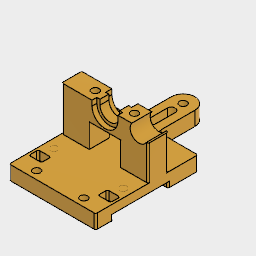
Extruder_Mount_F01 (Autodesk Fusion 360 design; units mm, degrees)
Autodesk Fusion 360 part; units mm, degrees
sketch "スケッチ1" plane through (0, 0, 0) normal (0, 0, 1) x (1, 0, 0)
  line L0 (27.5, 32.5) -> (-27.5, 32.5)
  line L1 (-27.5, 32.5) -> (-27.5, -32.5)
  line L2 (-27.5, -32.5) -> (27.5, -32.5)
  line L3 (27.5, -32.5) -> (27.5, 32.5)
  line L4 (27.5, 32.5) -> (-27.5, -32.5) construction
  line L5 (-27.5, 32.5) -> (27.5, -32.5) construction
  line L6 (-13, 32.5) -> (-13, 56.1)
  line L7 (-13, 56.1) -> (2, 56.1)
  line L8 (2, 56.1) -> (2, 32.5)
  circle A0 centre (-5.5, 56.1) radius 7.5
  line L9 (-5.5, 56.1) -> (-5.5, 32.5) construction
  circle A1 centre (-5.5, 36.1) radius 2.5
  circle A2 centre (-5.5, 48.6) radius 2.5
  line L10 (-3, 48.6) -> (-3, 36.1)
  line L11 (-8, 36.1) -> (-8, 48.6)
  line L12 (-27.5, 0.9) -> (27.5, 0.9)
  line L13 (27.5, 13.6) -> (-27.5, 13.6)
  dimension "d1" = 55
  dimension "d2" = 65
  dimension "d3" = 15
  dimension "d4" = 23.6
  dimension "d5" = 14.5
  dimension "d6" = 5
  dimension "d7" = 5
  dimension "d8" = 12.5
  dimension "d9" = 3.6
  dimension "d10" = 33.4
  dimension "d11" = 12.7
  measures "d1" distance of L1.end L2.end
  measures "d2" distance of L0.end L1.end
  measures "d3" distance of L6 L8
  measures "d4" distance of L0 L7
  measures "d5" distance of L1 L6
  measures "d6" diameter of A1
  measures "d7" diameter of A2
  measures "d8" distance of A1.centre A2.centre
  measures "d9" distance of L0 A1.centre
  measures "d10" distance of L2 L12
  measures "d11" distance of L12 L13
extrude "押し出し1" add sketch "スケッチ1" along normal blind 9 contours L0 L1 L3 L13 | L0 L6 L8 A0 A1 A2 L10 L11 | L1 L3 L12 L13 | L7 A0 A2 | L7 A0 | L1 L2 L3 L12
extrude "押し出し2" add sketch "スケッチ1" along normal blind 37 contours L1 L3 L12 L13
sketch "スケッチ2" plane through (0, 0, 0) normal (0, 0, -1) x (1, 0, 0)
  line L0 (-27.5, 32.5) -> (-27.5, -32.5)
  line L1 (-27.5, -32.5) -> (-13, -32.5)
  line L2 (-13, -32.5) -> (-13, -56.1)
  arc A0 (-13, -56.1) -> (2, -56.1) centre (-5.5, -56.1) ccw
  line L3 (2, -56.1) -> (2, -32.5)
  line L4 (2, -32.5) -> (27.5, -32.5)
  line L5 (27.5, -32.5) -> (27.5, 32.5)
  line L6 (27.5, 32.5) -> (-27.5, 32.5)
  arc A1 (-8, -48.6) -> (-3, -48.6) centre (-5.5, -48.6) ccw
  line L7 (-8, -48.6) -> (-8, -36.1)
  arc A2 (-3, -36.1) -> (-8, -36.1) centre (-5.5, -36.1) ccw
  line L8 (-3, -36.1) -> (-3, -48.6)
  line L9 (27.5, 21.5) -> (16.5, 21.5)
  line L10 (16.5, 21.5) -> (16.5, -13.5)
  line L11 (16.5, -13.5) -> (27.5, -13.5)
  line L12 (17.3, 6) -> (26.7, 6)
  line L13 (26.7, 6) -> (26.7, -6)
  line L14 (26.7, -6) -> (17.3, -6)
  line L15 (17.3, -6) -> (17.3, 6)
  line L16 (18, 21.5) -> (18, 15.5)
  line L17 (18, 15.5) -> (26, 15.5)
  line L18 (26, 15.5) -> (26, 21.5)
  circle A3 centre (22, 9.525) radius 2.35
  circle A4 centre (22, -9.525) radius 2.35
  line L19 (22, -13.5) -> (22, 21.5) construction
  line L20 (0, 32.5) -> (0, -32.5) construction
  line L21 (-16.5, -13.5) -> (-27.5, -13.5)
  line L22 (-16.5, 21.5) -> (-16.5, -13.5)
  line L23 (-27.5, 21.5) -> (-16.5, 21.5)
  line L24 (-18, 15.5) -> (-26, 15.5)
  line L25 (-18, 21.5) -> (-18, 15.5)
  line L26 (-26, 15.5) -> (-26, 21.5)
  circle A5 centre (-22, 9.525) radius 2.35
  line L27 (-17.3, 6) -> (-26.7, 6)
  line L28 (-26.7, 6) -> (-26.7, -6)
  line L29 (-17.3, -6) -> (-17.3, 6)
  line L30 (-26.7, -6) -> (-17.3, -6)
  circle A6 centre (-22, -9.525) radius 2.35
  circle A7 centre (0, 0) radius 2.35
  circle A8 centre (-12, -12) radius 1.5
  circle A9 centre (12, -12) radius 1.5
  circle A10 centre (12, 12) radius 1.5
  circle A11 centre (-12, 12) radius 1.5
  circle A12 centre (0, 0) radius 1.5
  dimension "d16" = 4.7
  dimension "d17" = 4.7
  dimension "d18" = 35
  dimension "d19" = 11
  dimension "d20" = 11
  dimension "d21" = 12
  dimension "d22" = 7.5
  dimension "d23" = 3.975
  dimension "d24" = 11.975
  dimension "d25" = 9.4
  dimension "d26" = 0.8
  dimension "d27" = 6
  dimension "d28" = 8
  dimension "d29" = 1.5
  dimension "d30" = 4.7
  dimension "d31" = 3
  dimension "d32" = 12
  dimension "d33" = 12
  dimension "d35" = 360
  dimension "d45" = 3
  measures "d16" diameter of A3
  measures "d17" diameter of A4
  measures "d18" distance of L9 L11
  measures "d19" distance of L6 L9
  measures "d20" distance of L10.end L11.end
  measures "d21" distance of L12.end L13.end
  measures "d22" distance of L11 L14
  measures "d23" distance of L11 A4.centre
  measures "d24" distance of L9 A3.centre
  measures "d25" distance of L13.end L14.end
  measures "d26" distance of L5 L13
  measures "d27" distance of L17.end L18.end
  measures "d28" distance of L16.end L17.end
  measures "d29" distance of L5 L18
  measures "d30" diameter of A7
  measures "d31" diameter of A8
  measures "d32" distance of A7.centre A8.centre
  measures "d33" distance of A7.centre A8.centre
  measures "d45" diameter of A12
extrude "押し出し3" cut sketch "スケッチ2" against normal through all contours L9 L16 L17 L18
extrude "押し出し4" cut sketch "スケッチ2" against normal blind 8.5 contours A3 | A4
extrude "押し出し5" cut sketch "スケッチ2" against normal blind 5 contours L12 L13 L14 L15
extrude "押し出し6" cut sketch "スケッチ2" against normal blind 3.5 contours L5 L9 L10 L11 L16 L17 L18
mirror "ミラー1" about plane through (0, 0, 0) normal (1, 0, 0) of "押し出し3", "押し出し4", "押し出し5", "押し出し6"
extrude "押し出し7" cut sketch "スケッチ2" against normal blind 8 contours A8 | A9 | A10 | A11
extrude "押し出し8" cut sketch "スケッチ2" against normal blind 8 contours A12
extrude "押し出し9" cut sketch "スケッチ2" against normal blind 5 contours A7
sketch "スケッチ3" plane through (0, 13.6, 0) normal (0, 1, 0) x (-1, 0, 0)
  line L0 (-27.5, 9) -> (27.5, 9)
  line L1 (27.5, 9) -> (27.5, 37)
  line L2 (27.5, 37) -> (-27.5, 37)
  line L3 (-27.5, 37) -> (-27.5, 9)
  line L4 (-10, 9) -> (-10, 24.2)
  line L5 (-10, 24.2) -> (10, 24.2)
  line L6 (10, 24.2) -> (10, 9)
  line L7 (0, 37) -> (0, 0) construction
  circle A0 centre (0, 33.75) radius 8.25
  circle A1 centre (0, 33.75) radius 6.25
  circle A2 centre (-21.5, 33.75) radius 5.5
  line L8 (6.25, 37) -> (6.25, 33.75)
  line L9 (-6.25, 37) -> (-6.25, 33.75)
  line L10 (8.25, 37) -> (8.25, 33.75)
  line L11 (-8.25, 37) -> (-8.25, 33.75)
  line L12 (-27.5, 31) -> (-26.2631, 31)
  line L13 (-27.5, 9) -> (-2, 9)
  line L14 (13, 9) -> (27.5, 9)
  circle A3 centre (10, 16.6) radius 1.25
  dimension "d50" = 16.5
  dimension "d51" = 12.5
  dimension "d52" = 11
  dimension "d53" = 3.25
  dimension "d54" = 6
  dimension "d55" = 3.25
  dimension "d56" = 22
  dimension "d57" = 20
  dimension "d58" = 17.5
  dimension "d59" = 15.2
  dimension "d60" = 2.5
  dimension "d61" = 7.6
  measures "d50" diameter of A0
  measures "d51" diameter of A1
  measures "d52" diameter of A2
  measures "d53" distance of L2 A0.centre
  measures "d54" distance of L3 A2.centre
  measures "d55" distance of L2 A2.centre
  measures "d56" distance of L12 L13
  measures "d57" distance of L4.end L5.end
  measures "d58" distance of L1 L6
  measures "d59" distance of L5.end L6.end
  measures "d60" diameter of A3
  measures "d61" distance of L0 A3.centre
extrude "押し出し10" cut sketch "スケッチ3" against normal through all contours L0 L4 L5 L6 L13 A3 | L6 A3 picked at (9.5938, 16.5073)
extrude "押し出し11" cut sketch "スケッチ3" against normal through all contours L2 A1 L9 | L2 A1 | L2 A1 L8 picked at (-0.4636, 33.8856)
extrude "押し出し12" cut sketch "スケッチ3" against normal through all from surface at -9.6 contours L2 A0 L11 | L2 A0 A1 L8 L9 | L2 A0 L10
extrude "押し出し13" cut sketch "スケッチ3" against normal blind 3.95 contours L2 A0 L11 | L2 A0 A1 L8 L9 | L2 A0 L10
extrude "押し出し14" cut sketch "スケッチ3" against normal through all contours L2 L3 A2 L12 | L2 A2 picked at (-22.8229, 31.257)
extrude "押し出し15" cut sketch "スケッチ3" against normal blind 4 contours L6 A3 picked at (10.7965, 16.3106)
sketch "スケッチ4" plane through (27.5, 0, 0) normal (1, 0, 0) x (0, 1, 0)
  line L0 (13.6, 31) -> (0.9, 31)
  line L1 (0.9, 31) -> (0.9, 9)
  line L2 (0.9, 9) -> (-32.5, 9)
  line L3 (-32.5, 9) -> (-32.5, 0)
  line L4 (-32.5, 0) -> (-21.5, 0)
  line L5 (-21.5, 0) -> (-21.5, 3.5)
  line L6 (-21.5, 3.5) -> (13.5, 3.5)
  line L7 (13.5, 3.5) -> (13.5, 0)
  line L8 (13.5, 0) -> (32.5, 0)
  line L9 (32.5, 0) -> (32.5, 9)
  line L10 (32.5, 9) -> (13.6, 9)
  line L11 (13.6, 9) -> (13.6, 31)
  circle A0 centre (13.6, 15.6) radius 1.25
  dimension "d71" = 2.5
  dimension "d72" = 6.6
  measures "d71" diameter of A0
  measures "d72" distance of L10.end A0.centre
extrude "押し出し16" cut sketch "スケッチ4" against normal blind 11 from surface at -3.5 contours L11 A0 picked at (13.1845, 15.9855)
sketch "スケッチ5" plane through (0, 0, 9) normal (0, 0, 1) x (-1, 0, 0)
  line L0 (-18, 15.5) -> (-26, 15.5)
  line L1 (-26, 15.5) -> (-26, 21.5)
  line L2 (-26, 21.5) -> (-18, 21.5)
  line L3 (-18, 21.5) -> (-18, 15.5)
  line L4 (27.5, -13.6) -> (10, -13.6)
  line L5 (10, -13.6) -> (10, -0.9)
  line L6 (10, -0.9) -> (27.5, -0.9)
  line L7 (27.5, -0.9) -> (27.5, 32.5)
  line L8 (27.5, 32.5) -> (-27.5, 32.5)
  line L9 (-27.5, 32.5) -> (-27.5, -0.9)
  line L10 (-27.5, -0.9) -> (-10, -0.9)
  line L11 (-10, -0.9) -> (-10, -13.6)
  line L12 (-10, -13.6) -> (-27.5, -13.6)
  line L13 (-27.5, -13.6) -> (-27.5, -32.5)
  line L14 (-27.5, -32.5) -> (-2, -32.5)
  line L15 (-2, -32.5) -> (-2, -56.1)
  arc A0 (-2, -56.1) -> (13, -56.1) centre (5.5, -56.1) ccw
  line L16 (13, -56.1) -> (13, -32.5)
  line L17 (13, -32.5) -> (27.5, -32.5)
  line L18 (27.5, -32.5) -> (27.5, -13.6)
  arc A1 (3, -48.6) -> (8, -48.6) centre (5.5, -48.6) ccw
  line L19 (3, -48.6) -> (3, -36.1)
  arc A2 (8, -36.1) -> (3, -36.1) centre (5.5, -36.1) ccw
  line L20 (8, -36.1) -> (8, -48.6)
  circle A3 centre (5.5, -56.1) radius 2.35
  circle A4 centre (5.5, -56.1) radius 1.75
  circle A5 centre (15, 27.5) radius 2.35
  circle A6 centre (15, 27.5) radius 1.75
  circle A7 centre (-15, 27.5) radius 2.35
  circle A8 centre (-15, 27.5) radius 1.75
  line L21 (18, 21.5) -> (26, 21.5)
  line L22 (26, 21.5) -> (26, 15.5)
  line L23 (26, 15.5) -> (18, 15.5)
  line L24 (18, 15.5) -> (18, 21.5)
  dimension "d76" = 4.7
  dimension "d77" = 3.5
  dimension "d78" = 4.7
  dimension "d79" = 3.5
  dimension "d80" = 4.7
  dimension "d81" = 3.5
  dimension "d82" = 5
  dimension "d83" = 12.5
  dimension "d84" = 12.5
  measures "d76" diameter of A3
  measures "d77" diameter of A4
  measures "d78" diameter of A5
  measures "d79" diameter of A6
  measures "d80" diameter of A7
  measures "d81" diameter of A8
  measures "d82" distance of L8 A5.centre
  measures "d83" distance of L7 A5.centre
  measures "d84" distance of L9 A7.centre
extrude "押し出し17" cut sketch "スケッチ5" against normal blind 8 contours A4 | A6 | A8
extrude "押し出し18" cut sketch "スケッチ5" against normal blind 5 contours A3 | A5 | A7
sketch "スケッチ6" plane through (0, 0, 37) normal (0, 0, 1) x (-1, 0, 0)
  line L0 (8.25, -9.65) -> (8.25, -13.6)
  line L1 (8.25, -13.6) -> (27.5, -13.6)
  line L2 (27.5, -13.6) -> (27.5, -0.9)
  line L3 (27.5, -0.9) -> (8.25, -0.9)
  line L4 (8.25, -0.9) -> (8.25, -4)
  line L5 (8.25, -4) -> (6.25, -4)
  line L6 (6.25, -4) -> (6.25, -9.65)
  line L7 (6.25, -9.65) -> (8.25, -9.65)
  line L8 (-27.5, -13.6) -> (-27.5, -0.9)
  line L9 (27.5, -7.25) -> (-27.5, -7.25) construction
  circle A0 centre (12.5, -7.25) radius 2.35
  circle A1 centre (12.5, -7.25) radius 1.75
  circle A2 centre (-12.5, -7.25) radius 2.35
  circle A3 centre (-12.5, -7.25) radius 1.75
  dimension "d89" = 4.7
  dimension "d90" = 4.7
  dimension "d91" = 3.5
  dimension "d92" = 3.5
  dimension "d93" = 15
  dimension "d94" = 15
  measures "d89" diameter of A0
  measures "d90" diameter of A2
  measures "d91" diameter of A3
  measures "d92" diameter of A1
  measures "d93" distance of L2 A0.centre
  measures "d94" distance of L8 A2.centre
extrude "押し出し19" cut sketch "スケッチ6" against normal blind 10 contours A1 | A3
extrude "押し出し20" cut sketch "スケッチ6" against normal blind 5 contours A0 | A2
fillet "フィレット1" radius 1 12 edges at (27.5, -32.5, 4.5) (27.5, -21.5, 1.75) (27.5, 13.5, 1.75) (27.5, 32.5, 4.5) (-27.5, 32.5, 4.5) (-27.5, -32.5, 4.5) (-27.5, 13.6, 23) (-27.5, 0.9, 23) (27.5, 0.9, 20) (27.5, 13.6, 20) (-27.5, 13.5, 1.75) (-27.5, -21.5, 1.75)
fillet "フィレット2" radius 1 8 edges at (18, -15.5, 6.25) (18, -21.5, 6.25) (26, -15.5, 6.25) (26, -21.5, 6.25) (-18, -21.5, 6.25) (-18, -15.5, 6.25) (-26, -15.5, 6.25) (-26, -21.5, 6.25)
fillet "フィレット3" radius 1 3 edges at (-11.25, 9.6, 16.6) (13, 12.35, 15.6) (24, 12.35, 15.6)
fillet "フィレット4" radius 2 2 edges at (2, 32.5, 4.5) (-13, 32.5, 4.5)
